test (Autodesk Fusion 360 design; units mm, degrees)
Autodesk Fusion 360 part; units mm, degrees
sketch "Sketch1" plane through (0, 0, 0) normal (1, 0, 0) x (0, 1, 0)
  line L0 (60, 70) -> (127.8158, 58.2135)
  line L1 (127.8158, 58.2135) -> (134.0564, 37.8275)
  line L2 (134.0564, 37.8275) -> (127.8158, 23.058)
  line L3 (127.8158, 23.058) -> (67.9154, 4.7211)
  line L4 (67.9154, 4.7211) -> (42.064, 15.6443)
  line L5 (42.064, 15.6443) -> (28.174, 36.9954)
  line L6 (28.174, 36.9954) -> (28.174, 52.8049)
  line L7 (28.174, 52.8049) -> (35.119, 64.8701)
  line L8 (35.119, 64.8701) -> (28.174, 68.8678)
  line L9 (28.174, 68.8678) -> (31.6465, 71.1268)
  line L10 (31.6465, 71.1268) -> (39.0435, 66.869)
  line L11 (39.0435, 66.869) -> (60, 70)
  constraint perpendicular L1 L3
  constraint perpendicular L2 L4
  constraint vertical L6
  constraint perpendicular L7 L8
  constraint perpendicular L5 L9
  constraint perpendicular L7 L10
extrude "Extrude1" add sketch "Sketch1" along normal blind 160
sketch "Sketch2" plane through (0, 13.5687, 78.0699) normal (0, 0.171235, 0.98523) x (-1, 0, 0)
  line L0 (0, -115.9598) -> (0, -47.1273)
  line L1 (0, -47.1273) -> (-160, -47.1273)
  line L2 (-160, -47.1273) -> (-160, -115.9598)
  line L3 (-160, -115.9598) -> (0, -115.9598)
  line L4 (-116.377, -61.3452) -> (-40, -61.3452)
  line L5 (-40, -61.3452) -> (-40, -90)
  line L6 (-40, -90) -> (-116.377, -90)
  line L7 (-116.377, -90) -> (-116.377, -61.3452)
  constraint horizontal L4
  constraint vertical L5
  constraint horizontal L6
  constraint vertical L7
extrude "Extrude2" add sketch "Sketch2" along normal blind 25 contours L4 L5 L6 L7
sketch "Sketch3" plane through (0, 17.8496, 102.7006) normal (0, 0.171235, 0.98523) x (-1, 0, 0)
  line L0 (-116.377, -90) -> (-40, -90)
  line L1 (-40, -90) -> (-40, -61.3452)
  line L2 (-40, -61.3452) -> (-116.377, -61.3452)
  line L3 (-116.377, -61.3452) -> (-116.377, -90)
  circle A0 centre (-85, -70) radius 5
extrude "Extrude3" add sketch "Sketch3" along normal blind 20 contours A0
sketch "Sketch4" plane through (0, 0, 0) normal (-1, 0, 0) x (0, -1, 0)
  line L0 (-31.6465, 71.1268) -> (-39.0435, 66.869)
  line L1 (-39.0435, 66.869) -> (-60, 70)
  line L2 (-60, 70) -> (-127.8158, 58.2135)
  line L3 (-127.8158, 58.2135) -> (-134.0564, 37.8275)
  line L4 (-134.0564, 37.8275) -> (-127.8158, 23.058)
  line L5 (-127.8158, 23.058) -> (-67.9154, 4.7211)
  line L6 (-67.9154, 4.7211) -> (-42.064, 15.6443)
  line L7 (-42.064, 15.6443) -> (-28.174, 36.9954)
  line L8 (-28.174, 36.9954) -> (-28.174, 52.8049)
  line L9 (-28.174, 52.8049) -> (-35.119, 64.8701)
  line L10 (-35.119, 64.8701) -> (-28.174, 68.8678)
  line L11 (-28.174, 68.8678) -> (-31.6465, 71.1268)
  circle A0 centre (-87.4582, 44.0936) radius 11.7609
extrude "Extrude4" add sketch "Sketch4" along normal blind 45 contours A0
